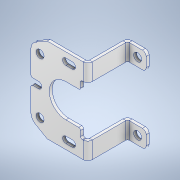
# Autodesk Inventor part: Idler Shear Brace
Saved by Autodesk Inventor 2020 (Build 240168000, 168)
## iProperties
Created: 2023-06-16
Part Number: Idler Shear Brace
Material: Aluminum 6061
Document SubType Name: Sheet Metal
Designer: Ishaan
Density: 2.7 g/cm^3
Appearance: Aluminum - Flat
Sheet Metal Rule: SendCutSend_Alu_1-16
Author: Ishaan
Autodesk Inventor part; units mm, degrees
ref_plane "YZ Plane" through (0, 0, 0) normal (1, 0, 0) x (0, 1, 0)
sketch "Sketch1" plane through (0, 0, 0) normal (0, 0, 1) x (1, 0, 0)
  line L0 (0, -15) -> (0, 15) construction
  line L1 (5, -15) -> (5, 15)
  line L2 (-5, 15) -> (-5, -15)
  arc A0 (-5, -15) -> (5, -15) centre (0, -15) ccw
  arc A1 (5, 15) -> (-5, 15) centre (0, 15) ccw
  line L3 (-2.5, 19.3301) -> (3.8564, 23)
  line L4 (3.8564, 23) -> (34, 23)
  line L5 (34, -23) -> (3.8564, -23)
  line L6 (3.8564, -23) -> (-2.5, -19.3301)
  line L7 (14, 0) -> (17.5, 0) construction
  line L8 (14, -9) -> (17.5, -9)
  line L9 (17.5, 9) -> (14, 9)
  arc A2 (14, 9) -> (14, -9) centre (14, 0) ccw
  arc A3 (17.5, -9) -> (17.5, 9) centre (17.5, 0) ccw
  line L10 (32.3848, 0) -> (14, 18.3848) construction
  line L11 (14, 18.3848) -> (-4.3848, 0) construction
  line L12 (-4.3848, 0) -> (14, -18.3848) construction
  line L13 (14, -18.3848) -> (32.3848, 0) construction
  line L14 (32.3848, 0) -> (-4.3848, 0) construction
  line L15 (14, 18.3848) -> (14, -18.3848) construction
  line L16 (-4.3848, 0) -> (-0.8848, 0) construction
  line L17 (-4.3848, -1.75) -> (-0.8848, -1.75)
  line L18 (-0.8848, 1.75) -> (-4.3848, 1.75)
  arc A4 (-4.3848, 1.75) -> (-4.3848, -1.75) centre (-4.3848, 0) ccw
  arc A5 (-0.8848, -1.75) -> (-0.8848, 1.75) centre (-0.8848, 0) ccw
  line L19 (14, 18.3848) -> (17.5, 18.3848) construction
  line L20 (14, 16.6348) -> (17.5, 16.6348)
  line L21 (17.5, 20.1348) -> (14, 20.1348)
  arc A6 (14, 20.1348) -> (14, 16.6348) centre (14, 18.3848) ccw
  arc A7 (17.5, 16.6348) -> (17.5, 20.1348) centre (17.5, 18.3848) ccw
  line L22 (14, -18.3848) -> (17.5, -18.3848) construction
  line L23 (14, -16.6348) -> (17.5, -16.6348)
  line L24 (17.5, -20.1348) -> (14, -20.1348)
  arc A8 (14, -16.6348) -> (14, -20.1348) centre (14, -18.3848) ccw
  arc A9 (17.5, -20.1348) -> (17.5, -16.6348) centre (17.5, -18.3848) ccw
  line L25 (32.3848, 0) -> (35.8848, 0) construction
  line L26 (32.3848, -1.75) -> (35.8848, -1.75)
  line L27 (35.8848, 1.75) -> (32.3848, 1.75)
  arc A10 (32.3848, 1.75) -> (32.3848, -1.75) centre (32.3848, 0) ccw
  arc A11 (35.8848, -1.75) -> (35.8848, 1.75) centre (35.8848, 0) ccw
  arc A12 (36, 21) -> (34, 23) centre (34, 21) ccw
  arc A13 (34, -23) -> (36, -21) centre (34, -21) ccw
  line L28 (14, 0) -> (17.5, 0) construction
  line L29 (14, -11.125) -> (17.5, -11.125) construction
  line L30 (17.5, 11.125) -> (14, 11.125) construction
  arc A14 (14, 11.125) -> (14, -11.125) centre (14, 0) ccw construction
  arc A15 (17.5, -11.125) -> (17.5, 11.125) centre (17.5, 0) ccw construction
  line L31 (34, -13.7696) -> (23, -13.7696)
  line L32 (22, -12.7696) -> (22, 12.7696)
  line L33 (23, 13.7696) -> (34, 13.7696)
  line L34 (22, 13.7696) -> (22, 23) construction
  line L35 (36, 21) -> (36, 15.7696)
  line L36 (36, -15.7696) -> (36, -21)
  arc A16 (34, 13.7696) -> (36, 15.7696) centre (34, 15.7696) ccw
  arc A17 (36, -15.7696) -> (34, -13.7696) centre (34, -15.7696) ccw
  arc A18 (23, 13.7696) -> (22, 12.7696) centre (23, 12.7696) ccw
  arc A19 (22, -12.7696) -> (23, -13.7696) centre (23, -12.7696) ccw
  line L37 (36, 23) -> (31.3848, 23) construction
  line L38 (31.3848, 23) -> (31.3848, 18.3848) construction
  line L39 (31.3848, 18.3848) -> (36, 18.3848) construction
  line L40 (36, 18.3848) -> (36, 23) construction
  line L41 (25.8848, 23) -> (25.8848, 13.7696)
  line L42 (25.8848, 18.3848) -> (31.3848, 18.3848) construction
  line L43 (25.8848, -13.7696) -> (25.8848, -23)
  line L44 (17.5, 9) -> (22, 9)
  line L45 (17.5, -9) -> (22, -9)
  point P0 (0, 0)
  point P1 (15.75, 0)
  point P2 (-2.6348, 0)
  point P3 (15.75, 18.3848)
  point P4 (15.75, -18.3848)
  point P5 (34.1348, 0)
  point P6 (15.75, 0)
  point P7 (22, 0)
  point P8 (22, 18.3848)
  point P9 (36, 18.3848)
  point P10 (31.3848, -18.3848)
  point P11 (25.8848, -18.3848)
  point P12 (-5, 1.6383)
  point P13 (-5, -1.6383)
  point P14 (22, -7.7942)
  point P15 (22, 7.7942)
  dimension "d0" = 15
  dimension "d1" = 10
  dimension "d3" = 46
  dimension "d4" = 120
  dimension "d5" = 120
  dimension "d6" = 17.5
  dimension "d7" = 18
  dimension "d8" = 3.5
  dimension "d9" = 26
  dimension "d11" = 1.75
  dimension "d12" = 2
  dimension "d13" = 22.25
  dimension "d15" = 36
  dimension "d16" = 2
  dimension "d17" = 1
  dimension "d18" = 14
  dimension "d19" = 5.5
  constraints: 106 end point, 45 tangent, 42 point on circle, 20 centre point, 16 midpoint, 14 parallel, 13 point on line, 12 perpendicular, 7 equal length, 6 equal radius, 4 collinear, 4 horizontal, 3 horizontal alignment, 2 vertical, 1 coincident, 1 vertical alignment
  measures "d0" distance of point (0, 0) L0.end
  measures "d1" diameter of A1
  measures "d3" distance between parallel lines of L5 L4
  measures "d4" angle of L2 L6
  measures "d5" angle of L3 L2
  measures "d6" distance from line of L0 L7.end
  measures "d7" distance between parallel lines of L8 L9
  measures "d8" distance of L9.start L9.end
  measures "d9" distance of L11.end L10.end
  measures "d11" radius of A4
  measures "d12" radius of A12
  measures "d13" diameter of A15
  measures "d15" distance between parallel lines of L35 L0
  measures "d16" radius of A16
  measures "d17" radius of A18
  measures "d18" distance between parallel lines of L35 L32
  measures "d19" distance of L42.start L42.end
extrude "Plate1" add sketch "Sketch1" along normal blind 1.6002 contours A0 L2 A4 L17 A5 L18 A1 L1 | L1 A2 L8 L45 L32 A19 L31 L43 L5 L6 A0 | L1 A1 L3 L4 L41 L33 A18 L32 L44 L9 A2 | A2 L9 A3 L32 L8 | L44 L32 A3 | A3 L32 L45 | L2 A4 L18 A5 L17 | A6 L21 A7 L20 | L23 A9 L24 A8
hole "Hole1" at (0, 15, 0) at (0, -15, 0) direction (0, 0, 1) diameter 4.3 end through all
extrude "Extrusion3" cut sketch "Sketch1" along normal through all contours A2 L9 A3 L32 L8 | L44 L32 A3 | A3 L32 L45 | L2 A4 L18 A5 L17 | A6 L21 A7 L20 | L23 A9 L24 A8
ref_plane "Work Plane2" through (0, 0, -21.6125) normal (0, 0, -1) x (-1, 0, 0)
sketch "Sketch3" plane through (24.2846, -23, 1.6002) normal (1, 0, 0) x (0, 1, 0)
  line L0 (9.2304, 0) -> (0, 0)
  line L1 (0, 0) -> (0, -23.2127)
  line L2 (0, -23.2127) -> (9.2304, -23.2127)
  line L3 (9.2304, -23.2127) -> (9.2304, 0)
  constraints: 6 end point, 1 horizontal, 1 perpendicular, 1 vertical
edge flange "Flange1" height 21.6125 angle 90 thickness 1.6002 bend radius 0.889 thickness toward (1, 0, 0) relief tear relief width 1.6002 relief depth 0.8001 corner gap 0.889 corner form 0 edges at (25.8848, -18.3848, 0) (25.8848, 18.3848, 0) wall of the first edge with corners at (24.2846, -13.7696, 1.6002) (24.2846, -23, 1.6002) (24.2846, -23, -21.6125) (24.2846, -13.7696, -21.6125)
bend "Bend1"
corner "Corner1"
sketch "Sketch4" plane through (24.2846, -13.7696, -20.0123) normal (0, 0, -1) x (-1, 0, 0)
  line L0 (0, -9.2304) -> (0, 0)
  line L1 (0, 0) -> (-13.6002, 0)
  line L2 (-13.6002, 0) -> (-13.6002, -9.2304)
  line L3 (-13.6002, -9.2304) -> (0, -9.2304)
  constraints: 6 end point, 1 horizontal, 1 perpendicular, 1 vertical
edge flange "Flange2" height 12 angle 90 thickness 1.6002 bend radius 0.889 thickness toward (0, 0, -1) relief tear relief width 1.6002 relief depth 0.8001 corner gap 0.889 corner form 0 edges at (25.8848, -18.3848, -21.6125) (25.8848, 18.3848, -21.6125) wall of the first edge with corners at (24.2846, -23, -20.0123) (24.2846, -13.7696, -20.0123) (37.8848, -13.7696, -20.0123) (37.8848, -23, -20.0123)
bend "Bend2"
corner "Corner2"
ref_plane "Work Plane1" through (0, 0, -21.6125) normal (0, 0, -1) x (-1, 0, 0)
sketch "Sketch5" plane through (37.8848, 13.7696, -20.0123) normal (0, 0, 1) x (1, 0, 0)
  line L0 (-11.111, 9.2304) -> (-11.111, 0) projected
  line L1 (-11.111, 0) -> (0, 0) projected
  line L2 (0, 0) -> (0, 9.2304) projected
  line L3 (-11.111, 9.2304) -> (0, 9.2304) projected
  line L4 (-11.111, -27.5391) -> (-11.111, -36.7696) projected
  line L5 (-11.111, -36.7696) -> (0, -36.7696) projected
  line L6 (0, -36.7696) -> (0, -27.5391) projected
  line L7 (-11.111, -27.5391) -> (0, -27.5391) projected
  line L8 (-1.8848, -29.5391) -> (-1.8848, -34.7696) projected
  line L9 (-1.8848, 7.2304) -> (-1.8848, 2) projected
  line L10 (-11.111, 9.2304) -> (0, 9.2304) projected
  line L11 (-1.8848, 9.2304) -> (-1.8848, 0)
  line L12 (-11.111, -27.5391) -> (0, -27.5391) projected
  line L13 (-1.8848, -27.5391) -> (-1.8848, -36.7696)
  line L14 (-11.111, -36.7696) -> (0, -36.7696) projected
  point P0 (-37.8848, -13.7696)
  point P1 (-1.8848, -29.5391)
  point P2 (-1.8848, -34.7696)
  point P3 (-1.8848, 7.2304)
  point P4 (-1.8848, 2)
  constraints: 4 end point, 4 point on line, 3 collinear, 1 perpendicular
extrude "Extrusion4" cut sketch "Sketch5" against normal through all contours L3 L2 L1 L11 L9 | L7 L6 L5 L13 L8
fillet "Fillet1" radius 2 4 edges at (36, -23, -20.8124) (36, -13.7696, -20.8124) (36, 13.7696, -20.8124) (36, 23, -20.8124)
fillet "Fillet2" radius 1 2 edges at (22, -9, 0.8001) (22, 9, 0.8001)
hole "Hole2" at (31.3848, 18.3848, 0) at (31.3848, -18.3848, 0) direction (0, 0, -1) diameter 4.3 end through all
fillet "Fillet3" radius 1 2 edges at (-5, 1.6383, 0.8001) (-5, -1.6383, 0.8001)
equation "\"d5\" = d4"
equation "\"d32\" = Thickness"
equation "\"d37\" = BendReliefWidth"
equation "\"d38\" = BendReliefDepth"
equation "\"d39\" = MinimumRemnant"
equation "\"d40\" = TransitionRadius"
equation "\"d43\" = BendRadius"
equation "\"d44\" = CornerReliefSize"
equation "\"d45\" = GapSize"
equation "\"d46\" = JacobiRadiusSize"
equation "\"d47\" = BendReliefWidth"
equation "\"d48\" = BendReliefDepth"
equation "\"d49\" = MinimumRemnant"
equation "\"d50\" = TransitionRadius"
equation "\"d53\" = BendRadius"
equation "\"d54\" = CornerReliefSize"
equation "\"d55\" = GapSize"
equation "\"d56\" = JacobiRadiusSize"
equation "\"BendReliefWidth\" = Thickness"
equation "\"BendReliefDepth\" = 0.5 * Thickness"
equation "\"CornerReliefSize\" = 4 * Thickness"
equation "\"MinimumRemnant\" = 2 * Thickness"
equation "\"TransitionRadius\" = BendRadius"
equation "\"JacobiRadiusSize\" = BendRadius"
equation "\"GapSize\" = Thickness"
equation "\"Thickness\" = 1.6002"
equation "\"BendRadius\" = 0.889"
body "Solid1"
